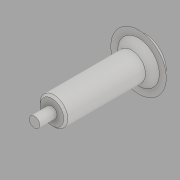
# Autodesk Inventor part: 2-2-2
Saved by Autodesk Inventor 2019 (Build 230136000, 136)
## iProperties
Created: 2020-11-06
Part Number: 2-2-2
Material: 一般
Document SubType Name: Modeling
Designer: Sugar
Density: 1 g/cm^3
Appearance: 預設
Author: Sugar
Autodesk Inventor part; units mm, degrees
ref_plane "YZ Plane" through (0, 0, 0) normal (1, 0, 0) x (0, 1, 0)
ref_plane "XZ Plane" through (0, 0, 0) normal (0, 1, 0) x (-1, 0, 0)
ref_plane "XY Plane" through (0, 0, 0) normal (0, 0, 1) x (1, 0, 0)
sketch "草圖1" plane through (0, 0, 0) normal (0, 0, 1) x (1, 0, 0)
  line L0 (0, 0) -> (0, 30)
  line L1 (-10, 30) -> (-20, 20)
  line L2 (-20, 20) -> (-132, 20)
  line L3 (-132, 20) -> (-135, 17)
  line L4 (-135, 17) -> (-135, 7.5)
  line L5 (-135, 7.5) -> (-160, 7.5)
  line L6 (-160, 7.5) -> (-160, 0)
  line L7 (-160, 0) -> (0, 0)
  line L8 (-10, 30) -> (-10, 40)
  line L9 (-10, 40) -> (0, 30)
  dimension "d3" = 45
  dimension "d4" = 150
  dimension "d5" = 7.5
  dimension "d6" = 25
  dimension "d7" = 45
  dimension "d8" = 3
  dimension "d9" = 20
  dimension "d10" = 160
  dimension "d11" = 40
  dimension "d12" = 10
  constraints: 20 end point, 2 parallel, 2 perpendicular, 2 vertical, 1 horizontal
  measures "d3" angle of L0 L9
  measures "d4" distance between parallel lines of L6 L8
  measures "d5" distance between parallel lines of L7 L5
  measures "d6" distance of L4.end L5.end
  measures "d7" angle of L4 L3
  measures "d8" horizontal distance of L2.end L3.end
  measures "d9" distance between parallel lines of L7 L2
  measures "d10" distance between parallel lines of L0 L6
  measures "d11" distance from line of L7 L8.end
  measures "d12" horizontal distance of L1.start L1.end
revolve "迴轉1" add sketch "草圖1" angle 360 about axis through (-160, 0, 0) along (1, 0, 0)
